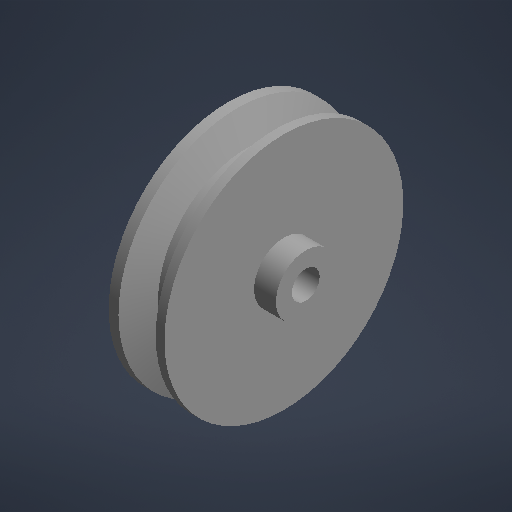
# Autodesk Inventor part: Rueda
Saved by Autodesk Inventor 2026.2 (Build 302298010, 298A)
## iProperties
Part Number: Rueda
Material: Generic
Document SubType Name: Modeling
Designer: diego
Appearance: Default
Author: diego
Autodesk Inventor part; units mm, degrees
ref_plane "YZ Plane" through (0, 0, 0) normal (1, 0, 0) x (0, 1, 0)
ref_plane "XZ Plane" through (0, 0, 0) normal (0, 1, 0) x (-1, 0, 0)
ref_plane "XY Plane" through (0, 0, 0) normal (0, 0, 1) x (1, 0, 0)
sketch "Sketch1" plane through (0, 0, 0) normal (1, 0, 0) x (0, 1, 0)
  circle A0 centre (0, 0) radius 60
  dimension "d0" = 120
  constraints: 1 centre point, 1 coincident
  measures "d0" diameter of A0
extrude "Extrusion1" add sketch "Sketch1" along normal blind 28
sketch "Sketch2" plane through (28, 0, 0) normal (1, 0, 0) x (0, 0, -1)
  circle A0 centre (0, 0) radius 7
  dimension "d3" = 14
  constraints: 1 centre point, 1 coincident
  measures "d3" diameter of A0
extrude "Extrusion2" cut sketch "Sketch2" against normal blind 28
sketch "Sketch3" plane through (0, 0, 0) normal (0, 1, 0) x (-1, 0, 0)
  line L0 (0, 60) -> (-28, 60) projected
  line L1 (-4.9193, 60) -> (-9.3746, 44.6454)
  line L2 (-9.3746, 44.6454) -> (-17.9139, 44.6454)
  line L3 (-17.9139, 44.6454) -> (-23.6686, 60)
  line L4 (-4.9193, 60) -> (-23.6686, 60)
  line L5 (-62.3987, 0) -> (62.1852, 0)
  point P0 (0, 0)
  constraints: 10 end point, 2 parallel, 2 point on line, 1 horizontal
revolve "Revolution1" cut sketch "Sketch3" angle 360 about axis through (62.3987, 0, 0) along (-1, 0, 0)
sketch "Sketch4" plane through (28, 0, 0) normal (1, 0, 0) x (0, 0, -1)
  circle A0 centre (0, 0) radius 15
  circle A1 centre (0, 0) radius 7
  dimension "d7" = 30
  dimension "d8" = 14
  constraints: 2 centre point, 2 coincident
  measures "d7" diameter of A0
  measures "d8" diameter of A1
extrude "Extrusion3" add sketch "Sketch4" along normal blind 11
sketch "Sketch5" plane through (0, 0, 0) normal (-1, 0, 0) x (0, 0, 1)
  circle A0 centre (0, 0) radius 7
  circle A1 centre (0, 0) radius 15
  dimension "d11" = 30
  dimension "d12" = 14
  constraints: 2 centre point, 2 coincident
  measures "d11" diameter of A1
  measures "d12" diameter of A0
extrude "Extrusion4" add sketch "Sketch5" along normal blind 11
body "Solid1"
